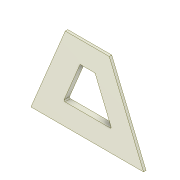
# Autodesk Inventor part: Stage2
Saved by Autodesk Inventor 2018.2 (Build 222227000, 227)
## iProperties
Created: 2018-11-01
Part Number: Stage2
Material: ABS-Kunststoff
Document SubType Name: Modeling
Designer: M.Knabel
Density: 1.06 g/cm^3
Appearance: Glatt - Elfenbein
Mass: 26.953 g
Surface Area: 131.178 cm^2
Volume: 25.4274 cm^3
Author: M.Knabel
Autodesk Inventor part; units mm, degrees
ref_plane "YZ Plane" through (0, 0, 0) normal (1, 0, 0) x (0, 1, 0)
ref_plane "XZ Plane" through (0, 0, 0) normal (0, 1, 0) x (-1, 0, 0)
ref_plane "XY Plane" through (0, 0, 0) normal (0, 0, 1) x (1, 0, 0)
sketch "Skizze1" plane through (0, 0, 0) normal (0, 1, 0) x (-1, 0, 0)
  line L0 (-22, 41.5) -> (22, 41.5)
  line L1 (22, 41.5) -> (56.3797, -41.5)
  line L2 (56.3797, -41.5) -> (-56.3797, -41.5)
  line L3 (-56.3797, -41.5) -> (-22, 41.5)
  line L4 (78.9316, 0) -> (-78.9316, 0) construction
  line L5 (0, -58.1) -> (0, 58.1) construction
  point P0 (0, 0)
  dimension "d0" = 83
  dimension "d1" = 112.5
  dimension "d2" = 44
  constraints: 8 end point, 1 horizontal, 1 parallel, 2 other
  measures "d0" distance between parallel lines of L2 L0
  measures "d1" angle of L0 L3
  measures "d2" distance of L0.start L0.end
extrude "Extrusion1" add sketch "Skizze1" along normal blind 6
sketch "Skizze2" plane through (0, 6, 0) normal (0, 1, 0) x (1, 0, 0)
  line L0 (-22, -41.5) -> (22, -41.5) projected
  line L1 (22, -41.5) -> (56.3797, 41.5) projected
  line L2 (56.3797, 41.5) -> (-56.3797, 41.5) projected
  line L3 (-56.3797, 41.5) -> (-22, -41.5) projected
  line L4 (-48.8967, 36.5) -> (48.8967, 36.5)
  line L5 (48.8967, 36.5) -> (18.6591, -36.5)
  line L6 (18.6591, -36.5) -> (-18.6591, -36.5)
  line L7 (-18.6591, -36.5) -> (-48.8967, 36.5)
  point P0 (0, 0)
  dimension "d5" = 5
  constraints: 8 end point, 3 other
  measures "d5" distance between parallel lines of L2 L4
extrude "Extrusion2" cut sketch "Skizze2" against normal blind 3.5
sketch "Skizze4" plane through (0, 6, 0) normal (0, 1, 0) x (1, 0, 0)
  line L0 (58.5766, 41.5) -> (-55.8797, 41.5) construction
  line L1 (-55.8797, 41.5) -> (-21.5, -41.5) construction
  line L2 (-21.5, -41.5) -> (24.1969, -41.5) construction
  line L3 (56.3797, 41.5) -> (22, -41.5) construction
  line L4 (22.4292, -40.7678) -> (56.8089, 42.2322) construction
  line L5 (-23.8211, 20.0791) -> (24.4471, 20.0791)
  line L6 (24.4471, 20.0791) -> (7.813, -20.0791)
  line L7 (7.813, -20.0791) -> (-7.187, -20.0791)
  line L8 (-7.187, -20.0791) -> (-23.8211, 20.0791)
  point P0 (0, 0)
  dimension "d15" = 15
  constraints: 8 end point, 3 other
  measures "d15" distance of L6.end L7.end
extrude "Extrusion3" cut sketch "Skizze4" against normal through all
fillet "Rundung1" radius 1 4 edges at (24.4471, 3, -20.0791) (7.813, 3, 20.0791) (-7.187, 3, 20.0791) (-23.8211, 3, -20.0791)
sketch "Skizze5" plane through (0, 6, 0) normal (0, 1, 0) x (1, 0, 0)
  line L0 (-7.4427, -19.4618) -> (-23.2484, 18.6965) projected
  arc A0 (-22.3245, 20.0791) -> (-23.2484, 18.6965) centre (-22.3245, 19.0791) ccw projected
  line L1 (-22.3245, 20.0791) -> (22.9504, 20.0791) projected
  arc A1 (23.8743, 18.6965) -> (22.9504, 20.0791) centre (22.9504, 19.0791) ccw projected
  line L2 (23.8743, 18.6965) -> (8.0687, -19.4618) projected
  arc A2 (7.1448, -20.0791) -> (8.0687, -19.4618) centre (7.1448, -19.0791) ccw projected
  line L3 (7.1448, -20.0791) -> (-6.5189, -20.0791) projected
  arc A3 (-7.4427, -19.4618) -> (-6.5189, -20.0791) centre (-6.5189, -19.0791) ccw projected
  line L4 (-48.8967, 36.5) -> (-18.6591, -36.5) projected
  line L5 (-18.6591, -36.5) -> (18.6591, -36.5) projected
  line L6 (18.6591, -36.5) -> (48.8967, 36.5) projected
  line L7 (48.8967, 36.5) -> (-48.8967, 36.5) projected
  point P0 (0, 0)
extrude "Extrusion4" cut sketch "Skizze5" against normal blind 0.5
